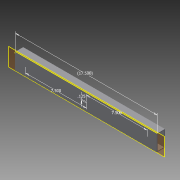
# Autodesk Inventor part: Drive base side
Saved by Autodesk Inventor 2015 (Build 190159000, 159)
## iProperties
Created: 2015-10-03
Part Number: Drive base side
Material: Generic
Document SubType Name: Modeling
Designer: alhohbein
Density: 1 g/cm^3
Appearance: Default
Author: alhohbein
Autodesk Inventor part; units mm, degrees
ref_plane "YZ Plane" through (0, 0, 0) normal (1, 0, 0) x (0, 1, 0)
ref_plane "XZ Plane" through (0, 0, 0) normal (0, 1, 0) x (-1, 0, 0)
sketch "Sketch1" plane through (0, 0, 0) normal (1, 0, 0) x (0, 1, 0)
  line L0 (2.54, 2.54) -> (-48.26, 2.54)
  line L1 (-48.26, 2.54) -> (-48.26, -22.86)
  line L2 (-48.26, -22.86) -> (2.54, -22.86)
  line L3 (2.54, -22.86) -> (2.54, 2.54)
  line L4 (0, 0) -> (-45.72, 0)
  line L5 (-45.72, 0) -> (-45.72, -20.32)
  line L6 (-45.72, -20.32) -> (0, -20.32)
  line L7 (0, -20.32) -> (0, 0)
  dimension "d0" = 50.8
  dimension "d1" = 25.4
  dimension "d5" = 2.54
  dimension "d6" = 2.54
  dimension "d7" = 2.54
  dimension "d8" = 2.54
  constraints: 16 end point, 6 perpendicular, 2 horizontal
  measures "d0" distance of L0.start L0.end
  measures "d1" distance of L2.end L0.start
  measures "d5" distance between parallel lines of L3 L7
  measures "d6" distance between parallel lines of L2 L6
  measures "d7" distance between parallel lines of L0 L4
  measures "d8" distance between parallel lines of L1 L5
extrude "Extrusion1" add sketch "Sketch1" along normal blind 444.5
ref_plane "Work Plane1" through (0, -48.26, 1.27) normal (0, 0, 1) x (1, 0, 0)
sketch "Sketch2" plane through (0, -48.26, 1.27) normal (0, 0, 1) x (1, 0, 0)
  line L0 (0, 50.8) -> (444.5, 50.8) projected
  line L1 (222.25, 50.8) -> (222.25, 0)
  line L2 (0, 0) -> (444.5, 0) projected
  line L3 (222.25, 25.4) -> (31.75, 25.4)
  line L4 (222.25, 25.4) -> (412.75, 25.4)
  line L5 (222.25, 25.4) -> (222.25, 22.225)
  point P0 (0, 48.26)
  dimension "d11" = 190.5
  dimension "d12" = 190.5
  dimension "d13" = 3.175
  dimension "d14" = 444.5
  constraints: 8 end point, 3 midpoint, 2 horizontal, 1 point on line
  measures "d11" distance of L3.start L3.end
  measures "d12" distance of L3.start L4.end
  measures "d13" distance of L3.start L5.end
  measures "d14" distance of L0.start L0.end
body "Solid1"
